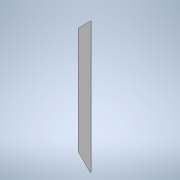
# Autodesk Inventor part: angle3
Saved by Autodesk Inventor 2020.1 (Build 241239000, 239)
## iProperties
Created: 2021-08-04
Part Number: angle3
Material: Generic
Document SubType Name: Modeling
Designer: Caleb
Density: 1 g/cm^3
Appearance: Default
Author: Caleb
Autodesk Inventor part; units mm, degrees
ref_plane "YZ Plane" through (0, 0, 0) normal (1, 0, 0) x (0, 1, 0)
ref_plane "XZ Plane" through (0, 0, 0) normal (0, 1, 0) x (-1, 0, 0)
ref_plane "XY Plane" through (0, 0, 0) normal (0, 0, 1) x (1, 0, 0)
sketch "Sketch1" plane through (0, 0, 0) normal (1, 0, 0) x (0, 1, 0)
  line L0 (-275, 24.5536) -> (275, 24.5536)
  line L1 (275, 24.5536) -> (275, -24.5536)
  line L2 (275, -24.5536) -> (-275, -24.5536)
  line L3 (-275, -24.5536) -> (-275, 24.5536)
  point P0 (0, 0)
  dimension "d15" = 550
  constraints: 8 end point, 2 parallel, 1 horizontal, 1 perpendicular
  measures "d15" distance of L1.end L2.end
extrude "Extrusion1" add sketch "Sketch1" along normal mid plane 50
sketch "Sketch2" plane through (-25, 275, 24.5536) normal (0, 1, 0) x (1, 0, 0)
  line L0 (50, 49.1071) -> (50, 0) projected
  line L1 (50, 4.1071) -> (5, 4.1071)
  line L2 (5, 4.1071) -> (5, 49.1071)
  line L3 (50, 49.1071) -> (0, 49.1071) projected
  line L4 (5, 49.1071) -> (50, 49.1071)
  line L5 (50, 49.1071) -> (50, 4.1071)
  point P0 (25, 24.5536)
  constraints: 8 end point, 3 perpendicular, 1 point on line
extrude "Extrusion2" cut sketch "Sketch2" against normal through all
sketch "Sketch5" plane through (-25, 0, 0) normal (-1, 0, 0) x (0, 0, 1)
  line L0 (-24.5536, 275) -> (-24.5536, -275) projected
  line L1 (20.4464, -275) -> (20.4464, 275) projected
  line L2 (-24.5536, 275) -> (20.4464, 275)
  line L3 (20.4464, 275) -> (20.4464, 225)
  line L4 (20.4464, 225) -> (-24.5536, 225)
  line L5 (-24.5536, 225) -> (-24.5536, 275)
  line L6 (-24.5536, -275) -> (24.5536, -275) projected
  line L7 (-24.5536, -275) -> (20.4464, -275)
  line L8 (20.4464, -275) -> (20.4464, -225)
  line L9 (20.4464, -225) -> (-24.5536, -225)
  line L10 (-24.5536, -225) -> (-24.5536, -275)
  point P0 (0, 0)
  constraints: 16 end point, 6 perpendicular, 2 point on line, 1 collinear
extrude "Extrusion5" cut sketch "Sketch5" against normal blind 10 contours L2 L1 L4 L0 | L9 L1 L6 L0
sketch "Sketch6" plane through (-25, -275, 24.5536) normal (0, 0, 1) x (1, 0, 0)
  line L0 (0, 500) -> (0, 50) projected
  line L1 (50, 0) -> (50, 550) projected
  line L2 (0, 500) -> (50, 550)
  line L3 (50, 550) -> (0, 550)
  line L4 (0, 550) -> (0, 500)
  line L5 (0, 50) -> (50, 0)
  line L6 (0, 0) -> (50, 0) projected
  line L7 (50, 0) -> (0, 0)
  line L8 (0, 0) -> (0, 50)
  point P0 (25, 275)
  constraints: 12 end point, 3 perpendicular, 1 horizontal
extrude "Extrusion6" cut sketch "Sketch6" against normal blind 5 contours L4 L3 L2 | L5 L6 L8
body "Solid1"
